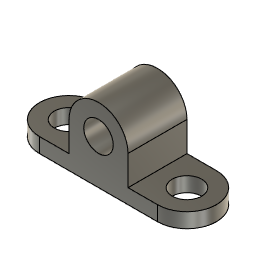
A4 (Autodesk Fusion 360 design; units mm, degrees)
Autodesk Fusion 360 part; units mm, degrees
sketch "Sketch1" plane through (0, 0, 0) normal (0, 0, 1) x (1, 0, 0)
  line L0 (40, -20) -> (-40, -20)
  line L1 (-40, 20) -> (40, 20)
  circle A0 centre (40, 0) radius 10
  circle A1 centre (-40, 0) radius 10
  arc A2 (40, -20) -> (40, 20) centre (40, 0) ccw
  arc A3 (-40, 20) -> (-40, -20) centre (-40, 0) ccw
  dimension "d1" = 80
  dimension "d2" = 40
  constraint horizontal L0
  constraint parallel L0 L1
  measures "d1" distance of L1.start L1.end
  measures "d2" distance of L0.end L1.start
extrude "Extrude1" add sketch "Sketch1" along normal blind 10
sketch "Sketch2" plane through (0, 0, 0) normal (0, 1, 0) x (1, 0, 0)
  line L0 (-20, -0.1094) -> (20, -0.1094)
  line L1 (20, -0.1094) -> (20, -30.1094)
  line L2 (-20, -30.1094) -> (-20, -0.1094)
  line L3 (-40, 0) -> (-40, -10)
  circle A0 centre (0, -30.1094) radius 20
  circle A1 centre (0, -30.1094) radius 10
  dimension "d9" = 40
  dimension "d10" = 30
  dimension "d11" = 20
  dimension "d12" = 40
  dimension "d13" = 20
  constraint horizontal L0
  constraint vertical L1
  constraint vertical L2
  constraint concentric A0 A1
  measures "d9" distance of L0.start L0.end
  measures "d10" distance of L0.start L2.start
  measures "d11" distance of L2 L3
  measures "d12" diameter of A0
  measures "d13" diameter of A1
extrude "Extrude2" add sketch "Sketch2" along normal mid plane 40
